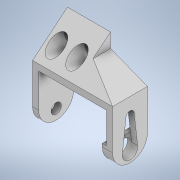
# Autodesk Inventor part: juncao8
Saved by Autodesk Inventor 2022.2 (Build 262287010, 287A)
## iProperties
Created: 2021-08-04
Part Number: juncao8
Material: Generic
Document SubType Name: Modeling
Designer: nakai
Density: 1 g/cm^3
Appearance: Default
Author: nakai
Autodesk Inventor part; units mm, degrees
ref_plane "YZ Plane" through (0, 0, 0) normal (1, 0, 0) x (0, 1, 0)
ref_plane "XZ Plane" through (0, 0, 0) normal (0, 1, 0) x (-1, 0, 0)
ref_plane "XY Plane" through (0, 0, 0) normal (0, 0, 1) x (1, 0, 0)
sketch "Sketch1" plane through (0, 0, 0) normal (0, 0, 1) x (1, 0, 0)
  line L0 (0, 0) -> (3, 0)
  line L1 (3, 0) -> (3, 25)
  line L2 (3, 25) -> (0, 25)
  line L3 (0, 25) -> (0, 0)
  line L4 (34, 25) -> (39, 25)
  line L5 (39, 25) -> (39, 0)
  line L6 (39, 0) -> (34, 0)
  line L7 (34, 0) -> (34, 25)
  line L8 (0, 25) -> (39, 25)
  line L9 (39, 25) -> (39, 42)
  line L10 (39, 42) -> (0, 42)
  line L11 (0, 42) -> (0, 25)
  line L12 (34, 25) -> (36, 25)
  line L13 (36, 25) -> (36, 10)
  line L14 (36, 10) -> (34, 10)
  line L15 (34, 10) -> (34, 25)
  point P0 (3, 25)
  point P1 (34, 25)
  dimension "d0" = 3
  dimension "d1" = 25
  dimension "d2" = 5
  dimension "d3" = 25
  dimension "d4" = 31
  dimension "d5" = 39
  dimension "d6" = 17
  dimension "d70" = 2
  dimension "d71" = 15
  constraints: 32 end point, 8 parallel, 4 horizontal, 4 perpendicular, 1 point on line
  measures "d0" distance of L2.end L1.end
  measures "d1" distance of L1.end L0.end
  measures "d2" distance of L5.end L6.end
  measures "d3" distance of L4.end L5.end
  measures "d4" distance between parallel lines of L7 L1
  measures "d5" distance of L10.end L9.end
  measures "d6" distance of L9.end L8.end
  measures "d70" distance of L13.end L14.end
  measures "d71" distance of L12.end L13.end
extrude "Extrusion1" add sketch "Sketch1" along normal blind 17 contours L3 L2 L1 L0 | L11 L10 L9 L4 L8 L2 | L4 L5 L6 L7 L14 L13
sketch "Sketch2" plane through (39, 0, 0) normal (1, 0, 0) x (0, 0, -1)
  line L0 (-17, 28) -> (-17, 42)
  line L1 (0, 42) -> (-17, 42) projected
  line L2 (-17, 42) -> (0, 42)
  line L3 (0, 42) -> (-17, 28)
  point P0 (0, 0)
  dimension "d9" = 14
  constraints: 6 end point, 1 perpendicular
  measures "d9" distance of L0.start L0.end
extrude "Extrusion2" cut sketch "Sketch2" against normal up to surface (39 mm away)
sketch "Sketch4" plane through (0, 0, 17) normal (0, 0, 1) x (1, 0, 0)
  line L0 (39, 0) -> (39, 42) projected
  line L1 (20, 42) -> (0, 42)
  line L2 (0, 42) -> (0, 25)
  line L3 (0, 25) -> (20, 25)
  line L4 (20, 25) -> (20, 42)
  circle A0 centre (15, 33.5) radius 3.5
  circle A1 centre (5, 33.5) radius 3.5
  line L5 (3, 25) -> (34, 25) projected
  line L6 (3, 25) -> (1, 25)
  point P0 (0, 0)
  dimension "d17" = 17
  dimension "d18" = 7
  dimension "d19" = 7
  dimension "d20" = 8.5
  dimension "d22" = 8.5
  dimension "d23" = 5
  dimension "d48" = 5
  dimension "d49" = 20
  constraints: 10 end point, 2 centre point, 2 horizontal, 2 parallel, 1 perpendicular
  measures "d17" distance of L1.end L2.end
  measures "d18" diameter of A0
  measures "d19" diameter of A1
  measures "d20" distance from line of L1 A0.centre
  measures "d22" distance from line of L1 A1.centre
  measures "d23" distance from line of L2 A1.centre
  measures "d48" distance from line of L4 A0.centre
  measures "d49" distance of L1.start L1.end
extrude "Extrusion4" cut sketch "Sketch4" against normal blind 14 contours A0 | A1
sketch "Sketch5" plane through (0, 0, 3) normal (0, 0, 1) x (1, 0, 0)
  arc A0 (15, 37) -> (15, 37) centre (15, 33.5) ccw projected
  circle A1 centre (15, 33.5) radius 1.5
  circle A2 centre (5, 33.5) radius 3.5 projected
  circle A3 centre (5, 33.5) radius 1.5
  point P0 (0, 0)
  point P1 (32.4191, 39.5294)
  point P2 (27.5809, 39.5294)
  point P3 (22.4191, 39.5294)
  point P4 (17.5809, 39.5294)
  dimension "d26" = 3
  dimension "d27" = 3
  constraints: 2 centre point, 2 coincident, 2 other
  measures "d26" diameter of A1
  measures "d27" diameter of A3
extrude "Extrusion5" cut sketch "Sketch5" against normal up to surface (3 mm away) contours A1 | A3
sketch "Sketch10" plane through (0, 0, 17) normal (0, 0, 1) x (1, 0, 0)
  line L0 (39, 42) -> (0, 42) projected
  line L1 (39, 42) -> (21, 42)
  line L2 (21, 42) -> (21, 35)
  line L3 (39, 28) -> (0, 28) projected
  line L4 (21, 35) -> (39, 28)
  line L5 (39, 42) -> (39, 28) projected
  line L6 (39, 28) -> (39, 42)
  point P0 (0, 0)
  dimension "d50" = 18
  dimension "d51" = 7
  constraints: 8 end point, 1 collinear, 1 perpendicular, 1 point on line
  measures "d50" distance of L0.start L1.end
  measures "d51" distance of L1.end L2.end
extrude "Extrusion10" cut sketch "Sketch10" against normal up to surface (17 mm away)
sketch "Sketch11" plane through (39, 0, 17) normal (1, 0, 0) x (0, 0, -1)
  circle A0 centre (8.5, 5) radius 3.75
  line L0 (17, 0) -> (0, 0) projected
  line L1 (17, 0) -> (17, 28) projected
  dimension "d54" = 7.5
  dimension "d55" = 5
  dimension "d56" = 8.5
  constraints: 1 centre point
  measures "d54" diameter of A0
  measures "d55" distance from line of L0 A0.centre
  measures "d56" distance from line of L1 A0.centre
extrude "Extrusion11" cut sketch "Sketch11" against normal up to surface (5 mm away)
sketch "Sketch12" plane through (0, 0, 0) normal (-1, 0, 0) x (0, 0, 1)
  circle A0 centre (8.5, 5) radius 2.5
  line L0 (0, 0) -> (17, 0) projected
  line L1 (17, 28) -> (17, 0) projected
  dimension "d59" = 5
  dimension "d60" = 5
  dimension "d61" = 8.5
  constraints: 1 centre point
  measures "d59" diameter of A0
  measures "d60" distance from line of L0 A0.centre
  measures "d61" distance from line of L1 A0.centre
extrude "Extrusion12" cut sketch "Sketch12" against normal up to surface (3 mm away)
fillet "Fillet2" radius 8.5 4 edges at (1.5, 0, 17) (1.5, 0, 0) (36.5, 0, 17) (36.5, 0, 0)
sketch "Sketch13" plane through (39, 28, 17) normal (1, 0, 0) x (0, 0, -1)
  circle A0 centre (8.5, -23) radius 3.75 projected
  circle A1 centre (8.5, -23) radius 3.5
  circle A2 centre (8.5, -8) radius 2
  circle A3 centre (8.5, -23) radius 3.75
  line L0 (10.4863, -7.7667) -> (12.2244, -22.5625)
  line L1 (6.5137, -7.7667) -> (4.7756, -22.5625)
  point P0 (17, -28)
  dimension "d65" = 4
  dimension "d66" = 15
  dimension "d67" = 0
  constraints: 4 end point, 4 point on circle, 4 tangent, 3 centre point, 1 coincident
  measures "d65" diameter of A2
  measures "d66" distance of A3.centre A2.centre
  measures "d67" horizontal distance of A3.centre A2.centre
extrude "Extrusion13" cut sketch "Sketch13" against normal blind 3 contours A0 | A0 L1 A2 L0 | A2 | A1
body "Solid1"
